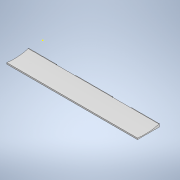
# Autodesk Inventor part: Pen Holder
Saved by Autodesk Inventor 2020.2 (Build 242310000, 310)
## iProperties
Created: 2020-05-07
Part Number: Pen Holder
Material: Generic
Document SubType Name: Modeling
Designer: Amaan Khalid
Density: 1 g/cm^3
Appearance: Default
Author: Amaan Khalid
Autodesk Inventor part; units mm, degrees
ref_plane "YZ Plane" through (0, 0, 0) normal (1, 0, 0) x (0, 1, 0)
ref_plane "XZ Plane" through (0, 0, 0) normal (0, 1, 0) x (-1, 0, 0)
ref_plane "XY Plane" through (0, 0, 0) normal (0, 0, 1) x (1, 0, 0)
sketch "Sketch1" plane through (0, 0, 0) normal (1, 0, 0) x (0, 1, 0)
  arc A0 (6.9666, 48.6647) -> (8.8296, 19.3623) centre (78.9029, 38.5279) ccw
  line L0 (6.9666, 48.6647) -> (5.1035, 48.6647)
  line L1 (5.1035, 48.6647) -> (5.1035, 18.7172)
  line L2 (5.1035, 18.7172) -> (8.8296, 18.7172)
  line L3 (8.8296, 18.7172) -> (8.8296, 19.3623)
  point P0 (0, 0)
  constraints: 8 end point, 2 horizontal, 2 perpendicular, 2 point on circle, 1 centre point
extrude "Extrusion1" add sketch "Sketch1" along normal blind 177.8
sketch "Sketch5" plane through (0, 8.8296, 19.3623) normal (0, 1, 0) x (1, 0, 0)
  point P0 (0, 19.3623)
sketch "Sketch6" plane through (0, 8.8296, 19.3623) normal (0, 1, 0) x (1, 0, 0)
  line L0 (0, 0.6451) -> (177.8, 0.6451) projected
  line L1 (38.1, 0.6451) -> (38.1, 0)
  line L2 (0, 0) -> (177.8, 0) projected
  line L3 (38.1, 0) -> (63.5, 0)
  line L4 (63.5, 0) -> (63.5, 0.6451)
  line L5 (63.5, 0.6451) -> (38.1, 0.6451)
  line L6 (114.3, 0.6451) -> (114.3, 0)
  line L7 (114.3, 0) -> (139.7, 0)
  line L8 (139.7, 0) -> (139.7, 0.6451)
  line L9 (114.3, 0.6451) -> (139.7, 0.6451)
  line L10 (0, 0.6451) -> (0, 0) projected
  point P0 (0, 19.3623)
  point P1 (63.5, 0)
  point P2 (63.5, 0.6451)
  dimension "d12" = 25.4
  dimension "d13" = 25.4
  dimension "d14" = 50.8
  dimension "d15" = 38.1
  constraints: 16 end point, 6 perpendicular, 6 point on line, 1 vertical
  measures "d12" distance of L1.end L3.end
  measures "d13" distance of L6.end L7.end
  measures "d14" distance between parallel lines of L6 L4
  measures "d15" distance between parallel lines of L1 L10
extrude "Extrusion4" cut sketch "Sketch6" against normal up to surface (1.863 mm away) contours L0 L4 L2 L1 | L0 L8 L2 L6
body "Solid1"
